Autodesk Inventor part; units mm, degrees
(part 2 of 3)
extrude "Выдавливание11" cut sketch "Эскиз1" against normal blind 6 contours A60 | A65
extrude "Выдавливание12" cut sketch "Эскиз1" against normal blind 4 contours L135 A107 L140 | A107 L135 | L135 A107 L136 L137 L138 L139 L140 | L140 A107 | L135 L136 A107 | A107 L139 L140 | A107 L136 | L139 A107 | L136 L137 A107 | A107 L138 L139 | A107 L137 | L138 A107 | L137 L138 A107 | A45 L144 A42 L143 L215 L141 | L215 A44 L142 A43 | L152 A108 L147 | A108 L152 L151 L150 L149 L148 L147 | L147 A108 | A108 L152 | A108 L148 L147 | L152 L151 A108 | L148 A108 | A108 L151 | A108 L149 L148 | L151 L150 A108 | L149 A108 | A108 L150 | A108 L150 L149 | L153 L219 L155 A46 L156 A49 | A47 L154 A48 L219 | A70 | A71
extrude "Выдавливание16" cut sketch "Эскиз1" against normal blind 2.5 contours L272 A86 L273 L60 L369 L368 L367 | L60 L66 L367 L372 A13 A85 L272 | A133 L72 L74 L73 L62 L280 | L280 A87 L279 A88 L278 A11 L71 L76 L75 L74 A133 | L60 L367 L66 | L62 L73 L78 L77 L278 A90 L277 A89 L280 | A13 L67 L372 L371 L370 A12 L273 A83 L267 L271 A85 | L291 A94 L290 L111 | L111 L290 A92 L289 A93 L292 A91 L291 | L71 L74 L72 | L367 L368 L369 L60 | L60 L369 L68 L370 L67 L372 L66 L367 | L66 L372 L367 | L72 L73 L62 | L66 L372 L67 | L322 A104 L328 A105 L329 A106 L321 L112 | L112 L321 A103 L322 | L74 L75 L76 L71 | L71 L76 L70 L77 L62 L73 L72 L74 | L72 L73 L74 | L60 L68 L369 | L273 A12 L68 L370 L369 L60 | L62 L77 L78 L73 | L67 L370 L371 L372 | L271 L117 L118 L119 L268 A84 L269 A81 L267 | L267 A83 L274 L122 L117 L271 | L71 L70 L76 | L369 L370 L68 | L77 L70 L62 | L370 L68 L67 | L271 L274 L262 L261 L260 L258 L257 L259 L122 L121 L268 L119 L118 L117 | L117 L122 L274 L259 L262 L271 | A11 L278 L62 L70 L77 L76 | L76 L77 L70 | L256 A82 L268 L121 L122 L274 | L274 L259 L257 L258 L260 L261 L262 | L262 L259 L274 | A10 | L116 L98 L115 L97 L251 A80 L252 A77 L250 A79 L239 A78 L95 | L95 L251 L97 L115 L98 L116 | A28 | A29 | A30 | A31 | A32 | A33 | A34 | A35 | L126 L127 L228 A75 L227 A73 L226 A74 L229 A72 L129 L130 L125 | L125 L130 L129 L228 L127 L126 | A38 | A39 | A50 | A51 | L160 L161 L162 L163 L164 L165 | L166 L167 L168 L169 L170 L171 | A52 L175 A53 L174 A54 L173 A55 L172 | A59 L181 A58 L180 A56 L179 A57 L178 | A60 | L187 L188 L189 L190 L191 L192 | A63 L196 A61 L195 A64 L194 A62 L193 | A69 L202 A66 L201 A67 L200 A68 L199 | A65 | L205 L206 L207 L208 L209 L210 | L220 L221 L222 L223 L224 L225 | L232 L234 L236 L235 L233 L231 | L237 L246 L247 L248 L249 L253 | L241 L243 L244 L245 L242 L240 | L254 L263 L264 L265 L266 L270 | L283 L284 L285 L286 L287 L288 | L298 A96 L304 A97 L305 A98 L297 A95 | L295 L299 L301 L306 L300 L296 | L310 A100 L316 A101 L317 A102 L309 A99 | L307 L311 L313 L318 L312 L308 | L319 L323 L325 L330 L324 L320 | A134
sketch "Эскиз3" plane through (0, 0, 4) normal (0, 0, 1) x (1, 0, 0)
  circle A0 centre (0, 55) radius 8 construction
  line L0 (-40.4221, -16.9869) -> (-34.9221, -26.5131)
  line L1 (-47.6314, -27.5) -> (0, 0) construction
  line L2 (-3, 128.25) -> (3, 128.25)
  line L3 (3, 128.25) -> (3, 122.2132)
  line L4 (-3, 122.2132) -> (-3, 128.25)
  line L5 (0, 63) -> (-54.5596, -31.5) construction
  line L6 (14, -6) -> (49, -6) construction
  line L7 (49, 6) -> (14, 6) construction
  line L8 (14, 6) -> (14, -6) construction
  line L9 (48.4771, 7.2527) -> (36.0246, 6.1632) construction
  line L10 (31, 11) -> (37, 11)
  line L11 (49, 1.2755) -> (48.4771, 7.2527) construction
  line L12 (49, 1.2755) -> (36.0246, 6.1632) construction
  line L13 (36.0246, 6.1632) -> (36.5476, 0.186) construction
  line L14 (36.5476, 0.186) -> (48.4771, 7.2527) construction
  line L15 (49, -2.1336) -> (36.5685, -0.827) construction
  line L16 (36.5685, -0.827) -> (35.9413, -6.7941) construction
  line L17 (35.9413, -6.7941) -> (48.3728, -8.1007) construction
  line L18 (49, 11) -> (19, 11)
  line L19 (0, 0) -> (63, 0) construction
  line L20 (14, -6) -> (49, 6) construction
  line L21 (49, -6) -> (14, 6) construction
  line L22 (19, -11) -> (49, -11)
  line L23 (37, -11) -> (31, -11)
  line L24 (48.3728, -8.1007) -> (36.5685, -0.827) construction
  circle A1 centre (0, -34.641) radius 20.7845 construction
  line L25 (31, -18) -> (37, -18)
  line L26 (37, -18) -> (37, -11)
  line L27 (31, -11) -> (31, -18)
  line L28 (54.5596, -31.5) -> (0, 63) construction
  circle A2 centre (0, 0) radius 55.4255 construction
  line L29 (-60.25, 121.25) -> (93.75, 121.25) construction
  line L30 (-60.25, 111.25) -> (93.75, 111.25) construction
  line L31 (-126.25, -126.25) -> (-126.25, 126.25)
  line L32 (-118.25, 74.25) -> (118.75, 74.25) construction
  line L33 (167.75, 130.25) -> (-130.25, 130.25)
  circle A3 centre (0, 0) radius 63
  line L34 (118.75, 59.25) -> (-118.25, 59.25) construction
  circle A4 centre (0, 0) radius 104
  circle A5 centre (0, 0) radius 110.3675
  line L35 (163.75, -126.25) -> (-126.25, -126.25)
  circle A6 centre (0, 0) radius 118.266 construction
  circle A7 centre (0, 0) radius 119.25
  line L36 (-130.25, -130.25) -> (167.75, -130.25)
  line L37 (-130.25, 130.25) -> (-130.25, -130.25)
  circle A8 centre (0, 0) radius 122.25
  line L38 (-126.25, 126.25) -> (163.75, 126.25)
  line L39 (163.75, 126.25) -> (163.75, -126.25)
  line L40 (-3, -128.25) -> (-3, -122.2132)
  line L41 (3, -128.25) -> (-3, -128.25)
  line L42 (3, -122.2132) -> (3, -128.25)
  line L43 (0, -128.25) -> (0, -119.25)
  line L44 (93, -126.25) -> (108, -126.25)
  circle A9 centre (93.75, -116.25) radius 5
  line L45 (-60.25, -111.25) -> (93.75, -111.25) construction
  line L46 (-60.25, -121.25) -> (93.75, -121.25) construction
  line L47 (-128.25, 3) -> (-128.25, -3)
  line L48 (-128.25, -3) -> (-122.2132, -3)
  line L49 (19, 11) -> (19, -11)
  line L50 (0, 0) -> (0, 14.85) construction
  line L51 (-49.5106, -37.2452) -> (-57.0106, -24.2548)
  circle A10 centre (-47.6314, -27.5) radius 2.5
  circle A11 centre (-38.7032, -26.9641) radius 1.5
  line L52 (-33.9221, -28.2452) -> (-57.0106, -24.2548) construction
  line L53 (-35.6542, -29.2452) -> (-49.5106, -37.2452)
  line L54 (167.75, -130.25) -> (167.75, 130.25)
  line L55 (-54.5596, -31.5) -> (54.5596, -31.5) construction
  line L56 (-126.25, -126.25) -> (-126.25, -130.25)
  line L57 (-122.2132, 3) -> (-128.25, 3)
  line L58 (-128.25, 0) -> (-119.25, 0)
  circle A12 centre (-118.25, 66.75) radius 7.5
  circle A13 centre (-42.7032, -20.0359) radius 1.5
  line L59 (-49.5106, -37.2452) -> (-41.4221, -15.2548) construction
  line L60 (-57.0106, -24.2548) -> (-43.1542, -16.2548)
  circle A14 centre (-47.6314, -27.5) radius 8 construction
  line L61 (-116.25, 101.25) -> (-70.25, 101.25) construction
  line L62 (163.75, 116.25) -> (163.75, 100.25)
  line L63 (0, -26.641) -> (0, -25.9661) construction
  circle A15 centre (93.75, 116.25) radius 5
  line L64 (35.6166, 11.7) -> (32.3834, 11.7)
  line L65 (32.3834, 11.7) -> (30.7668, 14.5)
  circle A16 centre (34, 14.5) radius 1.5
  line L66 (37.2332, 14.5) -> (35.6166, 11.7)
  line L67 (37, 11) -> (37, 18)
  arc A17 (37, 18) -> (49, 11) centre (49, 24.7857) ccw
  line L68 (35.9413, -6.7941) -> (49, -2.1336) construction
  line L69 (49, -6) -> (49, 6) construction
  line L70 (48.3728, -8.1007) -> (49, -2.1336) construction
  line L71 (49, -11) -> (49, 11)
  arc A18 (49, -11) -> (37, -18) centre (49, -24.7857) ccw
  circle A19 centre (34, -14.5) radius 1.5
  line L72 (32.3834, -17.3) -> (30.7668, -14.5)
  line L73 (32.3834, -11.7) -> (35.6166, -11.7)
  line L74 (35.6166, -11.7) -> (37.2332, -14.5)
  arc A20 (19, -11) -> (31, -18) centre (31, -4.2143) ccw
  line L75 (37.2332, -14.5) -> (35.6166, -17.3)
  line L76 (35.6166, -17.3) -> (32.3834, -17.3)
  line L77 (30.7668, -14.5) -> (32.3834, -11.7)
  line L78 (31, 18) -> (31, 11)
  arc A21 (31, 18) -> (19, 11) centre (31, 4.2143) ccw
  line L79 (37, 18) -> (31, 18)
  line L80 (32.3834, 17.3) -> (35.6166, 17.3)
  line L81 (35.6166, 17.3) -> (37.2332, 14.5)
  circle A22 centre (118.75, 66.75) radius 7.5
  line L82 (30.7668, 14.5) -> (32.3834, 17.3)
  line L83 (163.75, 126.25) -> (163.75, 130.25)
  line L84 (165.75, 116.25) -> (165.75, 100.25) construction
  line L85 (163.75, 100.25) -> (163.75, 116.25)
  line L86 (36.5476, 0.186) -> (49, 1.2755) construction
  line L87 (0, 0) -> (155.7962, -16.3748) construction
  line L88 (0, 0) -> (156.1718, 0) construction
  line L89 (0, 0) -> (156.3391, 13.6779) construction
  circle A23 centre (130, 40) radius 7.5
  line L90 (130, 47.5) -> (15, 47.5) construction
  line L91 (130, 32.5) -> (15, 32.5) construction
  line L92 (0, 128.25) -> (0, 119.25)
  circle A24 centre (15, 40) radius 7.5
  line L93 (-116.25, -126.25) -> (-70.25, -126.25) construction
  line L94 (-70.25, -106.25) -> (-116.25, -106.25) construction
  line L95 (-116.25, -106.25) -> (-116.25, -126.25) construction
  line L96 (-70.25, -126.25) -> (-70.25, -106.25) construction
  line L97 (-76, -126.25) -> (-61, -126.25)
  circle A25 centre (-60.25, -116.25) radius 5
  line L98 (162.25, -124.75) -> (162.25, -54.75)
  line L99 (112.25, -54.75) -> (112.25, -124.75)
  line L100 (162.25, -54.75) -> (112.25, -54.75)
  line L101 (163.75, -126.25) -> (163.75, -130.25)
  circle A26 centre (159.75, -122.75) radius 1.5
  circle A27 centre (159.75, -56.75) radius 1.5
  circle A28 centre (114.75, -56.75) radius 1.5
  line L102 (112.25, -124.75) -> (162.25, -124.75)
  line L103 (137.25, -89.75) -> (137.25, -86.8436) construction
  line L104 (137.25, -89.75) -> (144.2557, -89.75) construction
  line L105 (144.2557, -89.75) -> (137.25, -89.75) construction
  circle A29 centre (114.75, -122.75) radius 1.5
  line L106 (-126.25, 126.25) -> (-126.25, 130.25)
  line L107 (-70.25, 126.25) -> (-116.25, 126.25) construction
  line L108 (-70.25, 101.25) -> (-70.25, 126.25) construction
  line L109 (-116.25, 126.25) -> (-116.25, 101.25) construction
  circle A30 centre (-60.25, 116.25) radius 5
  circle A31 centre (15.5, -19.141) radius 1.75
  circle A32 centre (-15.5, -19.141) radius 1.75
  line L110 (0, -34.641) -> (5.9719, -34.641)
  line L111 (0, -34.641) -> (0, -30.5774)
  line L112 (21.15, -13.491) -> (-21.15, -13.491)
  circle A33 centre (-15.5, -50.141) radius 1.75
  line L113 (-21.15, -13.491) -> (-21.15, -55.791)
  line L114 (-21.15, -55.791) -> (21.15, -55.791)
  line L115 (21.15, -13.491) -> (-21.15, -55.791) construction
  line L116 (-21.15, -13.491) -> (21.15, -55.791) construction
  line L117 (21.15, -55.791) -> (21.15, -13.491)
  circle A34 centre (15.5, -50.141) radius 1.75
  line L118 (16.5, -13.491) -> (21.15, -18.141)
  line L119 (-16.5, -13.491) -> (-21.15, -18.141)
  line L120 (19, 11) -> (14, 11)
  line L121 (14, 11) -> (14, -11)
  line L122 (14, -11) -> (19, -11)
  line L123 (19, -11) -> (19, 11)
  line L124 (-43.1542, -16.2548) -> (-40.4221, -16.9869)
  line L125 (-35.6542, -29.2452) -> (-34.9221, -26.5131)
  line L126 (34.9221, -26.5131) -> (40.4221, -16.9869)
  line L127 (35.6542, -29.2452) -> (34.9221, -26.5131)
  line L128 (49.5106, -37.2452) -> (35.6542, -29.2452)
  line L129 (57.0106, -24.2548) -> (49.5106, -37.2452)
  line L130 (43.1542, -16.2548) -> (57.0106, -24.2548)
  line L131 (43.1542, -16.2548) -> (40.4221, -16.9869)
  circle A35 centre (42.7032, -20.0359) radius 1.5
  circle A36 centre (38.7032, -26.9641) radius 1.5
  circle A37 centre (47.6314, -27.5) radius 2.5
  circle A38 centre (47.6314, -27.5) radius 8 construction
  line L132 (57.0106, -24.2548) -> (33.9221, -28.2452) construction
  line L133 (41.4221, -15.2548) -> (49.5106, -37.2452) construction
  line L134 (5.5, 43.5) -> (-5.5, 43.5)
  line L135 (7.5, 45.5) -> (5.5, 43.5)
  line L136 (7.5, 61.5) -> (7.5, 45.5)
  line L137 (-7.5, 61.5) -> (7.5, 61.5)
  line L138 (-7.5, 45.5) -> (-7.5, 61.5)
  line L139 (-7.5, 45.5) -> (-5.5, 43.5)
  circle A39 centre (-4, 47) radius 1.5
  circle A40 centre (4, 47) radius 1.5
  circle A41 centre (0, 55) radius 2.5
  circle A42 centre (0, 55) radius 8 construction
  line L140 (-7.5, 61.5) -> (7.5, 43.5) construction
  line L141 (-7.5, 43.5) -> (7.5, 61.5) construction
  line L142 (165.75, 100.25) -> (163.75, 100.25) construction
  line L143 (165.75, 116.25) -> (163.75, 116.25) construction
  line L144 (163.75, -116.25) -> (163.75, -100.25)
  line L145 (165.75, -116.25) -> (163.75, -116.25) construction
  line L146 (165.75, -100.25) -> (163.75, -100.25) construction
  line L147 (165.75, -116.25) -> (165.75, -100.25) construction
  line L148 (163.75, -100.25) -> (163.75, -116.25)
  circle A43 centre (80, 17.5) radius 5.11 projected
  circle A44 centre (80, -17.5) radius 5.11 projected
  circle A45 centre (-80, -17.5) radius 5.11 projected
  circle A46 centre (-80, 17.5) radius 5.11 projected
  line L149 (87.95, 17.5) -> (87.95, -17.5) projected
  arc A47 (72.05, -17.5) -> (87.95, -17.5) centre (80, -17.5) ccw projected
  line L150 (72.05, -17.5) -> (72.05, 17.5) projected
  arc A48 (87.95, 17.5) -> (72.05, 17.5) centre (80, 17.5) ccw projected
  line L151 (-72.05, -17.5) -> (-72.05, 17.5) projected
  line L152 (-87.95, 17.5) -> (-87.95, -17.5) projected
  arc A49 (-72.05, 17.5) -> (-87.95, 17.5) centre (-80, 17.5) ccw projected
  arc A50 (-87.95, -17.5) -> (-72.05, -17.5) centre (-80, -17.5) ccw projected
  line L153 (-102.25, 70.75) -> (-108.25, 70.75) projected
  arc A51 (-102.25, 70.75) -> (-100.25, 72.75) centre (-102.25, 72.75) ccw projected
  line L154 (-100.25, 84.75) -> (-100.25, 72.75) projected
  arc A52 (-100.25, 84.75) -> (-102.25, 86.75) centre (-102.25, 84.75) ccw projected
  line L155 (-108.25, 86.75) -> (-102.25, 86.75) projected
  arc A53 (-102.25, -86.75) -> (-100.25, -84.75) centre (-102.25, -84.75) ccw projected
  line L156 (-108.25, -86.75) -> (-102.25, -86.75) projected
  line L157 (-100.25, -84.75) -> (-100.25, -72.75) projected
  arc A54 (-100.25, -72.75) -> (-102.25, -70.75) centre (-102.25, -72.75) ccw projected
  line L158 (-102.25, -70.75) -> (-108.25, -70.75) projected
  line L159 (-106.25, 84.75) -> (-106.25, 72.75) projected
  arc A55 (-106.25, 84.75) -> (-108.25, 86.75) centre (-108.25, 84.75) ccw projected
  line L160 (-120.25, 86.75) -> (-108.25, 86.75) projected
  arc A56 (-120.25, 86.75) -> (-122.25, 84.75) centre (-120.25, 84.75) ccw projected
  line L161 (-122.25, 72.75) -> (-122.25, 84.75) projected
  arc A57 (-122.25, 72.75) -> (-120.25, 70.75) centre (-120.25, 72.75) ccw projected
  line L162 (-108.25, 70.75) -> (-120.25, 70.75) projected
  arc A58 (-108.25, 70.75) -> (-106.25, 72.75) centre (-108.25, 72.75) ccw projected
  line L163 (-122.25, -84.75) -> (-122.25, -72.75) projected
  arc A59 (-122.25, -84.75) -> (-120.25, -86.75) centre (-120.25, -84.75) ccw projected
  line L164 (-108.25, -86.75) -> (-120.25, -86.75) projected
  arc A60 (-108.25, -86.75) -> (-106.25, -84.75) centre (-108.25, -84.75) ccw projected
  line L165 (-106.25, -72.75) -> (-106.25, -84.75) projected
  arc A61 (-106.25, -72.75) -> (-108.25, -70.75) centre (-108.25, -72.75) ccw projected
  line L166 (-120.25, -70.75) -> (-108.25, -70.75) projected
  arc A62 (-120.25, -70.75) -> (-122.25, -72.75) centre (-120.25, -72.75) ccw projected
  line L167 (-91.95, -17.5) -> (-91.95, 17.5)
  arc A63 (-68.05, 17.5) -> (-91.95, 17.5) centre (-80, 17.5) ccw
  line L168 (-68.05, 17.5) -> (-68.05, -17.5)
  arc A64 (-91.95, -17.5) -> (-68.05, -17.5) centre (-80, -17.5) ccw
  line L169 (68.05, 17.5) -> (68.05, -17.5)
  arc A65 (68.05, -17.5) -> (91.95, -17.5) centre (80, -17.5) ccw
  line L170 (91.95, -17.5) -> (91.95, 17.5)
  arc A66 (91.95, 17.5) -> (68.05, 17.5) centre (80, 17.5) ccw
  line L171 (140.75, -116.25) -> (136.75, -116.25) projected
  arc A67 (134.75, -114.25) -> (136.75, -116.25) centre (136.75, -114.25) ccw projected
  line L172 (134.75, -114.25) -> (134.75, -102.25) projected
  arc A68 (136.75, -100.25) -> (134.75, -102.25) centre (136.75, -102.25) ccw projected
  line L173 (136.75, -100.25) -> (140.75, -100.25) projected
  line L174 (142.75, -100.25) -> (140.75, -100.25) projected
  line L175 (154.75, -100.25) -> (142.75, -100.25) projected
  arc A69 (156.75, -102.25) -> (154.75, -100.25) centre (154.75, -102.25) ccw projected
  line L176 (156.75, -114.25) -> (156.75, -102.25) projected
  arc A70 (154.75, -116.25) -> (156.75, -114.25) centre (154.75, -114.25) ccw projected
  line L177 (142.75, -116.25) -> (154.75, -116.25) projected
  line L178 (142.75, -116.25) -> (140.75, -116.25) projected
  line L179 (154.75, 100.25) -> (142.75, 100.25) projected
  line L180 (142.75, 100.25) -> (140.75, 100.25) projected
  line L181 (136.75, 100.25) -> (140.75, 100.25) projected
  arc A71 (134.75, 102.25) -> (136.75, 100.25) centre (136.75, 102.25) ccw projected
  line L182 (134.75, 114.25) -> (134.75, 102.25) projected
  arc A72 (136.75, 116.25) -> (134.75, 114.25) centre (136.75, 114.25) ccw projected
  line L183 (140.75, 116.25) -> (136.75, 116.25) projected
  line L184 (142.75, 116.25) -> (140.75, 116.25) projected
  line L185 (142.75, 116.25) -> (154.75, 116.25) projected
  arc A73 (156.75, 114.25) -> (154.75, 116.25) centre (154.75, 114.25) ccw projected
  line L186 (156.75, 114.25) -> (156.75, 102.25) projected
  arc A74 (154.75, 100.25) -> (156.75, 102.25) centre (154.75, 102.25) ccw projected
  point P0 (-45.4663, -26.25)
  point P1 (42.5123, 3.7193)
  point P2 (34, 11)
  point P3 (31.5, 0)
  point P4 (34, -11)
  point P5 (31, -14.5)
  point P6 (0, 122.25)
  point P7 (0, -122.25)
  point P8 (-122.25, 0)
  point P9 (-45.4663, -26.25)
  point P10 (42.4707, -4.4638)
  point P11 (31, 14.5)
  point P12 (112.25, -89.75)
  point P13 (137.25, -124.75)
  point P14 (54.5596, -31.5)
  point P15 (45.4663, -26.25)
  point P16 (0, 63)
  point P17 (0, 52.5)
  point P18 (-108.25, -70.75)
  point P19 (-108.25, -86.75)
  point P20 (-108.25, 70.75)
  dimension "d239" = 16
  dimension "d185" = 236.532
  dimension "d186" = 238.5
  dimension "d187" = 290
  dimension "d188" = 3
  dimension "d189" = 6
  dimension "d190" = 4
  dimension "d191" = 208
  dimension "d192" = 220.735
  dimension "d193" = 126
  dimension "d194" = 4
  dimension "d195" = 2
  dimension "d196" = 2
  dimension "d197" = 2
  dimension "d198" = 25
  dimension "d199" = 46
  dimension "d200" = 20
  dimension "d201" = 10
  dimension "d202" = 10
  dimension "d203" = 10
  dimension "d204" = 10
  dimension "d205" = 110.851
  dimension "d206" = 5
  dimension "d207" = 6
  dimension "d211" = 41.569
  dimension "d212" = 12
  dimension "d213" = 35
  dimension "d214" = 6
  dimension "d215" = 12.5
  dimension "d216" = 5
  dimension "d217" = 3
  dimension "d218" = 5.6
  dimension "d219" = 7
  dimension "d220" = 6
  dimension "d222" = 10
  dimension "d223" = 10
  dimension "d224" = 52
  dimension "d225" = 45
  dimension "d226" = 15
  dimension "d227" = 40
  dimension "d228" = 15
  dimension "d229" = 15
  dimension "d230" = 115
  dimension "d231" = 70
  dimension "d232" = 50
  dimension "d233" = 42
  dimension "d234" = 63
  dimension "d235" = 3
  dimension "d236" = 1.5
  dimension "d240" = 4
  dimension "d241" = 18
  dimension "d242" = 15
  dimension "d243" = 3
  dimension "d244" = 2
  dimension "d245" = 2
  dimension "d246" = 5
  dimension "d247" = 237
  dimension "d248" = 42.3
  dimension "d249" = 3.5
  dimension "d250" = 31
  dimension "d251" = 31
  dimension "d252" = 33
  dimension "d253" = 30
  dimension "d254" = 5
  dimension "d255" = 22
  constraints: 308 end point, 42 centre point, 39 point on line, 31 perpendicular, 31 point on circle, 27 parallel, 23 midpoint, 22 vertical alignment, 21 horizontal, 16 tangent, 15 coincident, 13 equal length, 13 symmetric about line, 9 horizontal alignment, 7 vertical, 6 equal radius, 1 collinear, 145 other
  measures "d185" diameter of A6
  measures "d186" diameter of A7
  measures "d187" distance of L31.end L38.end
  measures "d189" distance between parallel lines of L4 L3
  measures "d190" distance between parallel lines of L38 L33
  measures "d191" diameter of A4
  measures "d192" diameter of A5
  measures "d193" diameter of A3
  measures "d194" distance from line of point (-122.25, 0) L31
  measures "d195" distance between parallel lines of L38 L2
  measures "d196" distance between parallel lines of L31 L47
  measures "d197" distance between parallel lines of L35 L41
  measures "d198" distance of L107.end L61.start
  measures "d199" distance of L108.end L107.end
  measures "d200" distance of L94.end L95.end
  measures "d201" distance between parallel lines of L31 L95
  measures "d202" distance between parallel lines of L31 L109
  measures "d203" diameter of A30
  measures "d204" diameter of A15
  measures "d205" diameter of A2
  measures "d206" angle of L88 L89
  measures "d207" angle of L88 L87
  measures "d211" diameter of A1
  measures "d212" distance of L6.end L7.start
  measures "d213" distance of L7.start L8.start
  measures "d214" distance of L11.start L14.end
  measures "d215" distance of L14.end L9.end
  measures "d216" distance between parallel lines of L7 L18
  measures "d217" diameter of A19
  measures "d218" distance between parallel lines of L73 L76
  measures "d219" distance of L23.end L25.start
  measures "d220" distance of L25.start L25.end
  measures "d222" distance from line of L108 A30.centre
  measures "d223" distance from line of L38 A30.centre
  measures "d224" distance between parallel lines of L38 L32
  measures "d225" distance from line of L39 A22.centre
  measures "d226" diameter of A24
  measures "d227" vertical distance of A4.centre A24.centre
  measures "d228" horizontal distance of A4.centre A24.centre
  measures "d229" diameter of A23
  measures "d230" distance of L91.start L91.end
  measures "d231" distance of L98.start L98.end
  measures "d232" distance of L98.end L99.start
  measures "d235" diameter of A29
  measures "d236" distance between parallel lines of L35 L102
  measures "d240" distance edge to line of A10 L51
  measures "d241" distance of L52.end L59.end
  measures "d242" distance of L59.end L52.start
  measures "d243" diameter of A13
  measures "d244" distance edge to line of A13 L0
  measures "d245" distance edge to line of A13 L60
  measures "d246" diameter of A10
  measures "d247" distance of L32.start L32.end
  measures "d248" distance of L114.start L114.end
  measures "d249" diameter of A34
  measures "d250" distance of A31.centre A34.centre
  measures "d251" distance of A32.centre A31.centre
  measures "d252" distance of L119.start L118.start
  measures "d253" distance between parallel lines of L49 L71
  measures "d254" distance between parallel lines of L121 L49
  measures "d255" distance of L22.end L18.start
extrude "Выдавливание17" cut sketch "Эскиз1" against normal through all contours A107 L135 | L135 A107 L136 L137 L138 L139 L140 | L140 A107 | A107 L136 | L139 A107 | A107 L137 | L138 A107 | A108 L152 L151 L150 L149 L148 L147 | L147 A108 | A108 L152 | L148 A108 | A108 L151 | L149 A108 | A108 L150 | A70 | A71
extrude "Выдавливание19" add sketch "Эскиз3" against normal blind 4 separate body contours L0 L125 L53 L51 L60 L124 | L4 L38 L106 L33 L83 L3 L2 | L2 L92 L38 L4 | L2 L3 L38 L92 | L38 L92 A8 L4 | L4 A8 L57 L31 L38 | L38 L3 A8 L92 | A8 L92 A7 L58 | L31 L57 L47 L48 L56 L36 L37 L33 L106 | L38 L39 L35 L42 A8 L3 | A8 L43 A7 L92 | A8 L58 L31 L57 | L31 L58 L47 L57 | L83 L33 L54 L36 L101 L39 | A7 | L58 A7 L43 A8 | A8 L48 L31 L58 | L31 L48 L47 L58 | A8 L40 L35 L31 L48 | L42 L35 L43 A8 | A8 L43 L35 L40 | L35 L40 L41 L42 L101 L36 L56 | L42 L41 L43 L35 | L35 L43 L41 L40 | L78 L65 L64 L66 L67 L10 | L10 L18 L71 L22 L49 | L18 A21 L78 L82 L65 | L67 L66 L81 A17 L18 | L49 L122 L121 L120 | L78 L82 L80 L81 L67 L66 L64 L65 | L65 L82 L78 | L67 L81 L66 | L22 L27 L77 L72 A20 L117 L112 | L79 L67 L81 L80 L82 L78 | A18 L26 L75 L74 L22 | L22 L26 L74 L73 L77 L27 | L112 L117 A20 | A20 L117 L118 L112 | L25 L27 L72 L76 L75 L26 | L77 L73 L74 L26 L75 L76 L72 L27 | L27 L72 L77 | L118 L117 L114 L113 L119 L112 | L74 L75 L26 | L119 L113 L112 | A3 | A4 | A5 | A9 | A10 | A11 | A12 L161 A57 L162 | L162 A57 L161 A12 | A12 L161 A56 L160 A55 L159 A58 L162 | A58 L159 A55 L155 A52 L154 A51 L153 | A13 | A15 | A16 | A19 | A22 | A23 | A24 | A25 | L102 L99 L100 L98 | A26 | A27 | A28 | A29 | A30 | A31 | A32 | A33 | A34 | L126 L131 L130 L129 L128 L127 | A35 | A36 | A37 | L134 L139 L138 L137 L136 L135 | A39 | A40 | A41 | A43 | A44 | A45 | A46 | L149 A47 L150 A48 | A50 L152 A49 L151 | L156 A60 L165 A61 L158 A54 L157 A53 | L164 A59 L163 A62 L166 A61 L165 A60 | L167 A63 L168 A64 | A66 L170 A65 L169 | L171 A67 L172 A68 L173 L174 L175 A69 L176 A70 L177 L178 | L179 L180 L181 A71 L182 A72 L183 L184 L185 A73 L186 A74
extrude "Выдавливание21" cut sketch "Эскиз3" against normal through all contours A43 | A44 | A45 | A46 | L149 A47 L150 A48 | A50 L152 A49 L151 bodies 2
extrude "Выдавливание22" cut sketch "Эскиз1" along normal blind 10 contours A6 | A7 | A10 | A15 | A16 | A17 | A18 | A19 | A20 | A21 | A22 | A23 | A24 | A28 | A29 | A30 | A31 | A32 | A33 | A34 | A35 | A38 | A39 | L135 A107 L140 | A107 L135 | L135 A107 L136 L137 L138 L139 L140 | L140 A107 | L135 L136 A107 | A107 L139 L140 | A107 L136 | L139 A107 | L136 L137 A107 | A107 L138 L139 | A107 L137 | L138 A107 | L137 L138 A107 | A45 L144 A42 L143 L215 L141 | L215 A44 L142 A43 | L152 A108 L147 | A108 L152 L151 L150 L149 L148 L147 | L147 A108 | A108 L152 | A108 L148 L147 | L152 L151 A108 | L148 A108 | A108 L151 | A108 L149 L148 | L151 L150 A108 | L149 A108 | A108 L150 | A108 L150 L149 | L153 L219 L155 A46 L156 A49 | A47 L154 A48 L219 | A50 | A51 | A60 | A65 | A70 | A71 | A134 bodies 2
extrude "Выдавливание23" cut sketch "Эскиз1" against normal blind 6 contours A30 | A31 | A32 | A33 bodies 1
extrude "Выдавливание24" cut sketch "Эскиз1" against normal up to surface (6 mm away) contours A10 | A21 | A22 | A23 | A24 | A28 | A29 | A34 | A35 | A38 | A39 | A50 | A51 | A134 bodies 1
extrude "Выдавливание27" cut sketch "Эскиз3" against normal blind 2 contours L167 A63 L168 A64 | A66 L170 A65 L169 bodies 2
extrude "Выдавливание30" cut sketch "Эскиз1" against normal through all contours A117 | A132 L342 | L342 A132 L343 L344 L345 L346 L347 | L347 A132 | A132 L343 | L346 A132 | A132 L344 | L345 A132 | A124 | A131 L363 L362 L361 L360 L359 L358 | L358 A131 | A131 L363 | L359 A131 | A131 L362 | L360 A131 | A131 L361 bodies 1
extrude "Выдавливание31" cut sketch "Эскиз1" against normal blind 4 contours L334 A121 L335 A120 L336 A123 L337 A122 | A117 | L342 A132 L347 | A132 L342 | L342 A132 L343 L344 L345 L346 L347 | L347 A132 | L342 L343 A132 | A132 L346 L347 | A132 L343 | L346 A132 | L343 L344 A132 | A132 L345 L346 | A132 L344 | L344 L345 A132 | L345 A132 | A129 L353 A130 L352 A127 L351 A128 L350 | A124 | L363 A131 L358 | A131 L363 L362 L361 L360 L359 L358 | L358 A131 | A131 L363 | A131 L359 L358 | L363 L362 A131 | L359 A131 | A131 L362 | A131 L360 L359 | L362 L361 A131 | L360 A131 | A131 L361 L360 | A131 L361 bodies 1
extrude "Выдавливание32" cut sketch "Эскиз1" along normal through all contours L334 A121 L335 A120 L336 A123 L337 A122 | A117 | L342 A132 L347 | A132 L342 | L342 A132 L343 L344 L345 L346 L347 | L347 A132 | L342 L343 A132 | A132 L346 L347 | A132 L343 | L346 A132 | L343 L344 A132 | A132 L345 L346 | A132 L344 | L344 L345 A132 | L345 A132 | A129 L353 A130 L352 A127 L351 A128 L350 | A124 | L363 A131 L358 | A131 L363 L362 L361 L360 L359 L358 | L358 A131 | A131 L363 | A131 L359 L358 | L363 L362 A131 | L359 A131 | A131 L362 | A131 L360 L359 | L362 L361 A131 | L360 A131 | A131 L361 L360 | A131 L361 bodies 2
extrude "Выдавливание33" cut sketch "Эскиз3" against normal blind 2 contours A58 L159 A55 L155 A52 L154 A51 L153 | L156 A60 L165 A61 L158 A54 L157 A53 | L171 A67 L172 A68 L173 L174 L175 A69 L176 A70 L177 L178 | L179 L180 L181 A71 L182 A72 L183 L184 L185 A73 L186 A74 bodies 2
sketch "Эскиз4" plane through (0, 0, 4) normal (0, 0, 1) x (1, 0, 0)
  circle A0 centre (0, 55) radius 8 construction
  line L0 (-40.4221, -16.9869) -> (-34.9221, -26.5131)
  line L1 (-47.6314, -27.5) -> (0, 0) construction
  line L2 (-3, 128.25) -> (3, 128.25)
  line L3 (3, 128.25) -> (3, 122.2132)
  line L4 (-3, 122.2132) -> (-3, 128.25)
  line L5 (0, 63) -> (-54.5596, -31.5) construction
  line L6 (14, -6) -> (49, -6) construction
  line L7 (49, 6) -> (14, 6) construction
  line L8 (14, 6) -> (14, -6) construction
  line L9 (48.4771, 7.2527) -> (36.0246, 6.1632) construction
  line L10 (31, 11) -> (37, 11)
  line L11 (49, 1.2755) -> (48.4771, 7.2527) construction
  line L12 (49, 1.2755) -> (36.0246, 6.1632) construction
  line L13 (36.0246, 6.1632) -> (36.5476, 0.186) construction
  line L14 (36.5476, 0.186) -> (48.4771, 7.2527) construction
  line L15 (49, -2.1336) -> (36.5685, -0.827) construction
  line L16 (36.5685, -0.827) -> (35.9413, -6.7941) construction
  line L17 (35.9413, -6.7941) -> (48.3728, -8.1007) construction
  line L18 (49, 11) -> (19, 11)
  line L19 (0, 0) -> (63, 0) construction
  line L20 (14, -6) -> (49, 6) construction
  line L21 (49, -6) -> (14, 6) construction
  line L22 (19, -11) -> (49, -11)
  line L23 (37, -11) -> (31, -11)
  line L24 (48.3728, -8.1007) -> (36.5685, -0.827) construction
  circle A1 centre (0, -34.641) radius 20.7845 construction
  line L25 (31, -18) -> (37, -18)
  line L26 (37, -18) -> (37, -11)
  line L27 (31, -11) -> (31, -18)
  line L28 (54.5596, -31.5) -> (0, 63) construction
  circle A2 centre (0, 0) radius 55.4255 construction
  line L29 (-70.25, 121.25) -> (93.75, 121.25) construction
  line L30 (-70.25, 111.25) -> (93.75, 111.25) construction
  line L31 (-126.25, -126.25) -> (-126.25, 126.25)
  line L32 (-117.25, 68.25) -> (118.75, 68.25) construction
  line L33 (167.75, 130.25) -> (-130.25, 130.25)
  circle A3 centre (0, 0) radius 63
  line L34 (118.75, 53.25) -> (-117.25, 53.25) construction
  circle A4 centre (0, 0) radius 104
  circle A5 centre (0, 0) radius 110.3675
  line L35 (163.75, -126.25) -> (-126.25, -126.25)
  circle A6 centre (0, 0) radius 118.266 construction
  circle A7 centre (0, 0) radius 119.25
  line L36 (-130.25, -130.25) -> (167.75, -130.25)
  line L37 (-130.25, 130.25) -> (-130.25, -130.25)
  circle A8 centre (0, 0) radius 122.25
  line L38 (-126.25, 126.25) -> (163.75, 126.25)
  line L39 (163.75, 126.25) -> (163.75, -126.25)
  line L40 (-3, -128.25) -> (-3, -122.2132)
  line L41 (3, -128.25) -> (-3, -128.25)
  line L42 (3, -122.2132) -> (3, -128.25)
  line L43 (0, -128.25) -> (0, -119.25)
  line L44 (93, -126.25) -> (108, -126.25)
  circle A9 centre (93.75, -116.25) radius 5
  line L45 (-70.25, -111.25) -> (93.75, -111.25) construction
  line L46 (-70.25, -121.25) -> (93.75, -121.25) construction
  line L47 (-128.25, 3) -> (-128.25, -3)
  line L48 (-128.25, -3) -> (-122.2132, -3)
  line L49 (19, 11) -> (19, -11)
  line L50 (0, 0) -> (0, 14.3794) construction
  line L51 (-49.5106, -37.2452) -> (-57.0106, -24.2548)
  circle A10 centre (-47.6314, -27.5) radius 2.5
  circle A11 centre (-38.7032, -26.9641) radius 1.5
  line L52 (-33.9221, -28.2452) -> (-57.0106, -24.2548) construction
  line L53 (-35.6542, -29.2452) -> (-49.5106, -37.2452)
  line L54 (167.75, -130.25) -> (167.75, 130.25)
  line L55 (-54.5596, -31.5) -> (54.5596, -31.5) construction
  line L56 (-126.25, -126.25) -> (-126.25, -130.25)
  line L57 (-122.2132, 3) -> (-128.25, 3)
  line L58 (-128.25, 0) -> (-119.25, 0)
  circle A12 centre (-117.25, 60.75) radius 7.5
  circle A13 centre (-42.7032, -20.0359) radius 1.5
  line L59 (-49.5106, -37.2452) -> (-41.4221, -15.2548) construction
  line L60 (-57.0106, -24.2548) -> (-43.1542, -16.2548)
  circle A14 centre (-47.6314, -27.5) radius 8 construction
  line L61 (-126.25, 101.25) -> (-80.25, 101.25)
  line L62 (163.75, 116.25) -> (163.75, 100.25)
  line L63 (0, -27.1116) -> (0, -26.4367) construction
  circle A15 centre (93.75, 116.25) radius 5
  line L64 (35.5588, 11.8) -> (32.4412, 11.8)
  line L65 (32.4412, 11.8) -> (30.8823, 14.5)
  circle A16 centre (34, 14.5) radius 1.5
  line L66 (37.1177, 14.5) -> (35.5588, 11.8)
  line L67 (37, 11) -> (37, 18)
  arc A17 (37, 18) -> (49, 11) centre (49, 24.7857) ccw
  line L68 (35.9413, -6.7941) -> (49, -2.1336) construction
  line L69 (49, -6) -> (49, 6) construction
  line L70 (48.3728, -8.1007) -> (49, -2.1336) construction
  line L71 (49, -11) -> (49, 11)
  arc A18 (49, -11) -> (37, -18) centre (49, -24.7857) ccw
  arc A19 (19, -11) -> (31, -18) centre (31, -4.2143) ccw
  line L72 (31, 18) -> (31, 11)
  arc A20 (31, 18) -> (19, 11) centre (31, 4.2143) ccw
  line L73 (37, 18) -> (31, 18)
  line L74 (32.4412, 17.2) -> (35.5588, 17.2)
  line L75 (35.5588, 17.2) -> (37.1177, 14.5)
  circle A21 centre (118.75, 60.75) radius 7.5
  line L76 (30.8823, 14.5) -> (32.4412, 17.2)
  line L77 (163.75, 126.25) -> (163.75, 130.25)
  line L78 (163.75, 100.25) -> (163.75, 116.25)
  line L79 (36.5476, 0.186) -> (49, 1.2755) construction
  line L80 (0, 0) -> (155.7962, -16.3748) construction
  line L81 (0, 0) -> (156.4435, 0) construction
  line L82 (0, 0) -> (156.3391, 13.6779) construction
  circle A22 centre (135, 40) radius 7.5
  line L83 (135, 47.5) -> (25, 47.5) construction
  line L84 (135, 32.5) -> (25, 32.5) construction
  line L85 (0, 128.25) -> (0, 119.25)
  circle A23 centre (25, 40) radius 7.5
  line L86 (-126.25, -126.25) -> (-80.25, -126.25)
  line L87 (-80.25, -101.25) -> (-126.25, -101.25)
  line L88 (-126.25, -101.25) -> (-126.25, -126.25)
  line L89 (-80.25, -126.25) -> (-80.25, -101.25)
  line L90 (-76, -126.25) -> (-61, -126.25)
  circle A24 centre (-70.25, -116.25) radius 5
  line L91 (162.25, -124.75) -> (162.25, -54.75)
  line L92 (112.25, -54.75) -> (112.25, -124.75)
  line L93 (162.25, -54.75) -> (112.25, -54.75)
  line L94 (163.75, -126.25) -> (163.75, -130.25)
  circle A25 centre (159.75, -122.75) radius 1.5
  circle A26 centre (159.75, -56.75) radius 1.5
  circle A27 centre (114.75, -56.75) radius 1.5
  line L95 (112.25, -124.75) -> (162.25, -124.75)
  line L96 (137.25, -89.75) -> (137.25, -87.3142) construction
  line L97 (137.25, -89.75) -> (144.5274, -89.75) construction
  line L98 (144.5274, -89.75) -> (137.25, -89.75) construction
  circle A28 centre (114.75, -122.75) radius 1.5
  line L99 (-126.25, 126.25) -> (-126.25, 130.25)
  line L100 (-80.25, 126.25) -> (-126.25, 126.25)
  line L101 (-80.25, 101.25) -> (-80.25, 126.25)
  line L102 (-126.25, 126.25) -> (-126.25, 101.25)
  circle A29 centre (-70.25, 116.25) radius 5
  circle A30 centre (15.5, -19.141) radius 1.5
  circle A31 centre (-15.5, -19.141) radius 1.5
  line L103 (0, -34.641) -> (5.9719, -34.641)
  line L104 (0, -34.641) -> (0, -31.0481)
  line L105 (21.15, -13.491) -> (-21.15, -13.491)
  circle A32 centre (-15.5, -50.141) radius 1.5
  line L106 (-21.15, -13.491) -> (-21.15, -55.791)
  line L107 (-21.15, -55.791) -> (21.15, -55.791)
  line L108 (21.15, -13.491) -> (-21.15, -55.791) construction
  line L109 (-21.15, -13.491) -> (21.15, -55.791) construction
  line L110 (21.15, -55.791) -> (21.15, -13.491)
  circle A33 centre (15.5, -50.141) radius 1.5
  line L111 (16.5, -13.491) -> (21.15, -18.141)
  line L112 (-16.5, -13.491) -> (-21.15, -18.141)
  line L113 (19, 11) -> (14, 11)
  line L114 (14, 11) -> (14, -11)
  line L115 (14, -11) -> (19, -11)
  line L116 (19, -11) -> (19, 11)
  line L117 (-43.1542, -16.2548) -> (-40.4221, -16.9869)
  line L118 (-35.6542, -29.2452) -> (-34.9221, -26.5131)
  line L119 (34.9221, -26.5131) -> (40.4221, -16.9869)
  line L120 (35.6542, -29.2452) -> (34.9221, -26.5131)
  line L121 (49.5106, -37.2452) -> (35.6542, -29.2452)
  line L122 (57.0106, -24.2548) -> (49.5106, -37.2452)
  line L123 (43.1542, -16.2548) -> (57.0106, -24.2548)
  line L124 (43.1542, -16.2548) -> (40.4221, -16.9869)
  circle A34 centre (42.7032, -20.0359) radius 1.5
  circle A35 centre (38.7032, -26.9641) radius 1.5
  circle A36 centre (47.6314, -27.5) radius 2.5
  circle A37 centre (47.6314, -27.5) radius 8 construction
  line L125 (57.0106, -24.2548) -> (33.9221, -28.2452) construction
  line L126 (41.4221, -15.2548) -> (49.5106, -37.2452) construction
  line L127 (5.5, 43.5) -> (-5.5, 43.5)
  line L128 (7.5, 45.5) -> (5.5, 43.5)
  line L129 (7.5, 61.5) -> (7.5, 45.5)
  line L130 (-7.5, 61.5) -> (7.5, 61.5)
  line L131 (-7.5, 45.5) -> (-7.5, 61.5)
  line L132 (-7.5, 45.5) -> (-5.5, 43.5)
  circle A38 centre (-4, 47) radius 1.5
  circle A39 centre (4, 47) radius 1.5
  circle A40 centre (0, 55) radius 2.5
  circle A41 centre (0, 55) radius 8 construction
  line L133 (-7.5, 61.5) -> (7.5, 43.5) construction
  line L134 (-7.5, 43.5) -> (7.5, 61.5) construction
  line L135 (163.75, -116.25) -> (163.75, -100.25)
  line L136 (163.75, -100.25) -> (163.75, -116.25)
  line L137 (-109.3, 75.8921) -> (-114.25, 73.0342)
  line L138 (-114.25, 73.0342) -> (-119.2, 75.8921)
  line L139 (-119.2, 75.8921) -> (-119.2, 81.6079)
  line L140 (-119.2, 81.6079) -> (-114.25, 84.4658)
  line L141 (-114.25, 84.4658) -> (-109.3, 81.6079)
  line L142 (-109.3, 81.6079) -> (-109.3, 75.8921)
  line L143 (-120.25, 70.75) -> (-108.25, 70.75)
  line L144 (-106.25, 72.75) -> (-106.25, 84.75)
  line L145 (-108.25, 86.75) -> (-120.25, 86.75)
  line L146 (-122.25, 84.75) -> (-122.25, 72.75)
  line L147 (-122.25, 70.75) -> (-106.25, 86.75) construction
  line L148 (-106.25, 70.75) -> (-122.25, 86.75) construction
  arc A42 (-120.25, 86.75) -> (-122.25, 84.75) centre (-120.25, 84.75) ccw
  arc A43 (-108.25, 70.75) -> (-106.25, 72.75) centre (-108.25, 72.75) ccw
  arc A44 (-106.25, 84.75) -> (-108.25, 86.75) centre (-108.25, 84.75) ccw
  arc A45 (-122.25, 72.75) -> (-120.25, 70.75) centre (-120.25, 72.75) ccw
  arc A46 (-122.25, -84.75) -> (-120.25, -86.75) centre (-120.25, -84.75) ccw
  line L149 (-119.2, -75.8921) -> (-119.2, -81.6079)
  line L150 (-109.3, -81.6079) -> (-109.3, -75.8921)
  line L151 (-119.2, -81.6079) -> (-114.25, -84.4658)
  line L152 (-114.25, -84.4658) -> (-109.3, -81.6079)
  line L153 (-108.25, -86.75) -> (-120.25, -86.75)
  line L154 (-114.25, -73.0342) -> (-119.2, -75.8921)
  line L155 (-109.3, -75.8921) -> (-114.25, -73.0342)
  line L156 (-122.25, -84.75) -> (-122.25, -72.75)
  arc A47 (-120.25, -70.75) -> (-122.25, -72.75) centre (-120.25, -72.75) ccw
  line L157 (-120.25, -70.75) -> (-108.25, -70.75)
  line L158 (-106.25, -70.75) -> (-122.25, -86.75) construction
  line L159 (-122.25, -70.75) -> (-106.25, -86.75) construction
  arc A48 (-106.25, -72.75) -> (-108.25, -70.75) centre (-108.25, -72.75) ccw
  line L160 (-106.25, -72.75) -> (-106.25, -84.75)
  arc A49 (-108.25, -86.75) -> (-106.25, -84.75) centre (-108.25, -84.75) ccw
  line L161 (-126.25, 101.25) -> (-80.25, 101.25)
  circle A50 centre (-114.75, 95.75) radius 1.5
  circle A51 centre (-91.75, 95.75) radius 1.5
  line L162 (-112.05, 97.3088) -> (-112.05, 94.1912)
  line L163 (-112.05, 94.1912) -> (-114.75, 92.6323)
  line L164 (-114.75, 92.6323) -> (-117.45, 94.1912)
  line L165 (-117.45, 94.1912) -> (-117.45, 97.3088)
  line L166 (-117.45, 97.3088) -> (-114.75, 98.8677)
  line L167 (-114.75, 98.8677) -> (-112.05, 97.3088)
  line L168 (-91.75, 98.8677) -> (-89.05, 97.3088)
  line L169 (-89.05, 97.3088) -> (-89.05, 94.1912)
  line L170 (-89.05, 94.1912) -> (-91.75, 92.6323)
  line L171 (-91.75, 92.6323) -> (-94.45, 94.1912)
  line L172 (-94.45, 94.1912) -> (-94.45, 97.3088)
  line L173 (-94.45, 97.3088) -> (-91.75, 98.8677)
  line L174 (-117.5, 91) -> (-112, 91)
  line L175 (-110, 93) -> (-110, 98.5)
  line L176 (-112, 100.5) -> (-117.5, 100.5)
  line L177 (-119.5, 98.5) -> (-119.5, 93)
  line L178 (-119.5, 91) -> (-110, 100.5) construction
  line L179 (-110, 91) -> (-119.5, 100.5) construction
  line L180 (-89, 100.5) -> (-94.5, 100.5)
  line L181 (-96.5, 98.5) -> (-96.5, 93)
  line L182 (-94.5, 91) -> (-89, 91)
  line L183 (-87, 93) -> (-87, 98.5)
  line L184 (-87, 100.5) -> (-96.5, 91) construction
  line L185 (-96.5, 100.5) -> (-87, 91) construction
  arc A52 (-119.5, 93) -> (-117.5, 91) centre (-117.5, 93) ccw
  arc A53 (-117.5, 100.5) -> (-119.5, 98.5) centre (-117.5, 98.5) ccw
  arc A54 (-110, 98.5) -> (-112, 100.5) centre (-112, 98.5) ccw
  arc A55 (-112, 91) -> (-110, 93) centre (-112, 93) ccw
  arc A56 (-96.5, 93) -> (-94.5, 91) centre (-94.5, 93) ccw
  arc A57 (-94.5, 100.5) -> (-96.5, 98.5) centre (-94.5, 98.5) ccw
  arc A58 (-89, 91) -> (-87, 93) centre (-89, 93) ccw
  arc A59 (-87, 98.5) -> (-89, 100.5) centre (-89, 98.5) ccw
  line L186 (-126.25, -101.25) -> (-80.25, -101.25)
  line L187 (-80.25, -101.25) -> (-80.25, -100.25)
  line L188 (-90.25, -90.25) -> (-116.25, -90.25)
  circle A60 centre (-91.75, -95.75) radius 1.5
  line L189 (-91.75, -92.6323) -> (-89.05, -94.1912)
  line L190 (-89.05, -94.1912) -> (-89.05, -97.3088)
  line L191 (-89.05, -97.3088) -> (-91.75, -98.8677)
  line L192 (-91.75, -98.8677) -> (-94.45, -97.3088)
  line L193 (-94.45, -97.3088) -> (-94.45, -94.1912)
  line L194 (-94.45, -94.1912) -> (-91.75, -92.6323)
  line L195 (-94.5, -100.5) -> (-89, -100.5)
  line L196 (-87, -98.5) -> (-87, -93)
  line L197 (-89, -91) -> (-94.5, -91)
  line L198 (-96.5, -93) -> (-96.5, -98.5)
  line L199 (-96.5, -100.5) -> (-87, -91) construction
  line L200 (-87, -100.5) -> (-96.5, -91) construction
  arc A61 (-94.5, -91) -> (-96.5, -93) centre (-94.5, -93) ccw
  arc A62 (-89, -100.5) -> (-87, -98.5) centre (-89, -98.5) ccw
  arc A63 (-96.5, -98.5) -> (-94.5, -100.5) centre (-94.5, -98.5) ccw
  arc A64 (-87, -93) -> (-89, -91) centre (-89, -93) ccw
  line L201 (-117.5, -100.5) -> (-112, -100.5)
  line L202 (-110, -98.5) -> (-110, -93)
  line L203 (-112, -91) -> (-117.5, -91)
  line L204 (-119.5, -93) -> (-119.5, -98.5)
  line L205 (-119.5, -100.5) -> (-110, -91) construction
  line L206 (-110, -100.5) -> (-119.5, -91) construction
  circle A65 centre (-114.75, -95.75) radius 1.5
  line L207 (-112.05, -94.1912) -> (-112.05, -97.3088)
  line L208 (-112.05, -97.3088) -> (-114.75, -98.8677)
  line L209 (-114.75, -98.8677) -> (-117.45, -97.3088)
  line L210 (-117.45, -97.3088) -> (-117.45, -94.1912)
  line L211 (-117.45, -94.1912) -> (-114.75, -92.6323)
  line L212 (-114.75, -92.6323) -> (-112.05, -94.1912)
  line L213 (-126.25, -100.25) -> (-126.25, -101.25)
  arc A66 (-117.5, -91) -> (-119.5, -93) centre (-117.5, -93) ccw
  arc A67 (-110, -93) -> (-112, -91) centre (-112, -93) ccw
  arc A68 (-112, -100.5) -> (-110, -98.5) centre (-112, -98.5) ccw
  arc A69 (-119.5, -98.5) -> (-117.5, -100.5) centre (-117.5, -98.5) ccw
  line L214 (-108.25, 86.75) -> (-102.25, 86.75)
  line L215 (-100.25, 84.75) -> (-100.25, 72.75)
  line L216 (-102.25, 70.75) -> (-108.25, 70.75)
  line L217 (-108.25, 70.75) -> (-108.25, 86.75)
  line L218 (-108.25, -86.75) -> (-102.25, -86.75)
  line L219 (-100.25, -84.75) -> (-100.25, -72.75)
  line L220 (-102.25, -70.75) -> (-108.25, -70.75)
  line L221 (-108.25, -70.75) -> (-108.25, -86.75)
  circle A70 centre (-114.25, 78.75) radius 3
  circle A71 centre (-114.25, -78.75) radius 3
  arc A72 (-9.7, 44.25) -> (-7.7, 42.25) centre (-7.7, 44.25) ccw
  line L222 (6.7, 45.4412) -> (4, 43.8823)
  line L223 (6.7, 48.5588) -> (6.7, 45.4412)
  line L224 (-7.7, 42.25) -> (7.7, 42.25)
  line L225 (9.7, 44.25) -> (9.7, 49.75)
  line L226 (4, 43.8823) -> (1.3, 45.4412)
  line L227 (4, 50.1177) -> (6.7, 48.5588)
  arc A73 (9.7, 49.75) -> (7.7, 51.75) centre (7.7, 49.75) ccw
  line L228 (1.3, 45.4412) -> (1.3, 48.5588)
  line L229 (-9.7, 49.75) -> (-9.7, 44.25)
  line L230 (1.3, 48.5588) -> (4, 50.1177)
  arc A74 (-7.7, 51.75) -> (-9.7, 49.75) centre (-7.7, 49.75) ccw
  line L231 (7.7, 51.75) -> (-7.7, 51.75)
  arc A75 (7.7, 42.25) -> (9.7, 44.25) centre (7.7, 44.25) ccw
  line L232 (0, 42.25) -> (0, 44.9705) construction
  line L233 (-4, 50.1177) -> (-6.7, 48.5588)
  line L234 (-6.7, 45.4412) -> (-4, 43.8823)
  line L235 (-6.7, 48.5588) -> (-6.7, 45.4412)
  line L236 (-1.3, 45.4412) -> (-1.3, 48.5588)
  line L237 (-4, 43.8823) -> (-1.3, 45.4412)
  line L238 (-1.3, 48.5588) -> (-4, 50.1177)
  circle A76 centre (-4, 47) radius 1.5
  line L239 (-42.7032, -16.9182) -> (-40.0032, -18.4771)
  arc A77 (-40.4396, -14.4566) -> (-43.1716, -13.7246) centre (-42.1716, -15.4566) ccw
  line L240 (-36.5896, -21.125) -> (-38.9456, -22.4853) construction
  arc A78 (-40.9668, -32.5434) -> (-38.2348, -33.2754) centre (-39.2348, -31.5434) ccw
  line L241 (-38.2348, -33.2754) -> (-33.4716, -30.5254)
  line L242 (-38.7032, -30.0818) -> (-36.0032, -28.5229)
  arc A79 (-33.4716, -30.5254) -> (-32.7396, -27.7934) centre (-34.4716, -28.7934) ccw
  line L243 (-41.4032, -28.5229) -> (-38.7032, -30.0818)
  line L244 (-36.0032, -28.5229) -> (-36.0032, -25.4053)
  line L245 (-41.4032, -25.4053) -> (-41.4032, -28.5229)
  line L246 (-38.7032, -23.8464) -> (-41.4032, -25.4053)
  line L247 (-36.0032, -25.4053) -> (-38.7032, -23.8464)
  line L248 (-40.0032, -18.4771) -> (-40.0032, -21.5947)
  line L249 (-40.0032, -21.5947) -> (-42.7032, -23.1536)
  line L250 (-42.7032, -23.1536) -> (-45.4032, -21.5947)
  line L251 (-45.4032, -21.5947) -> (-45.4032, -18.4771)
  line L252 (-32.7396, -27.7934) -> (-40.4396, -14.4566)
  line L253 (-48.6668, -19.2066) -> (-40.9668, -32.5434)
  arc A80 (-47.9348, -16.4746) -> (-48.6668, -19.2066) centre (-46.9348, -18.2066) ccw
  line L254 (-43.1716, -13.7246) -> (-47.9348, -16.4746)
  line L255 (-45.4032, -18.4771) -> (-42.7032, -16.9182)
  line L256 (36.0032, -28.5229) -> (36.0032, -25.4053)
  arc A81 (32.7396, -27.7934) -> (33.4716, -30.5254) centre (34.4716, -28.7934) ccw
  line L257 (36.5896, -21.125) -> (38.9456, -22.4853) construction
  arc A82 (48.6668, -19.2066) -> (47.9348, -16.4746) centre (46.9348, -18.2066) ccw
  line L258 (47.9348, -16.4746) -> (43.1716, -13.7246)
  line L259 (45.4032, -18.4771) -> (42.7032, -16.9182)
  arc A83 (43.1716, -13.7246) -> (40.4396, -14.4566) centre (42.1716, -15.4566) ccw
  line L260 (45.4032, -21.5947) -> (45.4032, -18.4771)
  line L261 (42.7032, -16.9182) -> (40.0032, -18.4771)
  line L262 (42.7032, -23.1536) -> (45.4032, -21.5947)
  line L263 (40.0032, -21.5947) -> (42.7032, -23.1536)
  line L264 (40.0032, -18.4771) -> (40.0032, -21.5947)
  line L265 (36.0032, -25.4053) -> (38.7032, -23.8464)
  line L266 (38.7032, -23.8464) -> (41.4032, -25.4053)
  line L267 (41.4032, -25.4053) -> (41.4032, -28.5229)
  line L268 (41.4032, -28.5229) -> (38.7032, -30.0818)
  line L269 (40.4396, -14.4566) -> (32.7396, -27.7934)
  line L270 (40.9668, -32.5434) -> (48.6668, -19.2066)
  arc A84 (38.2348, -33.2754) -> (40.9668, -32.5434) centre (39.2348, -31.5434) ccw
  line L271 (33.4716, -30.5254) -> (38.2348, -33.2754)
  line L272 (38.7032, -30.0818) -> (36.0032, -28.5229)
  line L273 (37.9143, -22.8306) -> (26.5604, -16.2754)
  line L274 (25.8284, -13.5434) -> (29.0857, -7.9015)
  line L275 (31.8178, -7.1694) -> (43.1716, -13.7246)
  line L276 (43.1716, -13.7246) -> (37.9143, -22.8306)
  line L277 (37.9143, -22.8306) -> (30.0857, -6.1694) construction
  line L278 (24.8284, -15.2754) -> (43.1716, -13.7246) construction
  line L279 (34, -14.5) -> (37.8782, -16.7391) construction
  line L280 (34, -14.5) -> (34.9387, -12.8741) construction
  line L281 (30.8823, -14.5) -> (32.4412, -11.8)
  line L282 (32.4412, -11.8) -> (35.5588, -11.8)
  line L283 (35.5588, -11.8) -> (37.1177, -14.5)
  line L284 (37.1177, -14.5) -> (35.5588, -17.2)
  line L285 (35.5588, -17.2) -> (32.4412, -17.2)
  line L286 (32.4412, -17.2) -> (30.8823, -14.5)
  circle A85 centre (34, -14.5) radius 1.5
  arc A86 (25.8284, -13.5434) -> (26.5604, -16.2754) centre (27.5604, -14.5434) ccw
  arc A87 (31.8178, -7.1694) -> (29.0857, -7.9015) centre (30.8178, -8.9015) ccw
  line L287 (31.25, 9.75) -> (36.75, 9.75)
  line L288 (38.75, 11.75) -> (38.75, 17.25)
  line L289 (36.75, 19.25) -> (31.25, 19.25)
  line L290 (29.25, 17.25) -> (29.25, 11.75)
  line L291 (29.25, 9.75) -> (38.75, 19.25) construction
  line L292 (38.75, 9.75) -> (29.25, 19.25) construction
  arc A88 (31.25, 19.25) -> (29.25, 17.25) centre (31.25, 17.25) ccw
  arc A89 (38.75, 17.25) -> (36.75, 19.25) centre (36.75, 17.25) ccw
  arc A90 (29.25, 11.75) -> (31.25, 9.75) centre (31.25, 11.75) ccw
  arc A91 (36.75, 9.75) -> (38.75, 11.75) centre (36.75, 11.75) ccw
  arc A92 (12.75, -14.391) -> (10.75, -16.391) centre (12.75, -16.391) ccw
  line L293 (12.8, -17.5822) -> (15.5, -16.0233)
  line L294 (12.8, -20.6998) -> (12.8, -17.5822)
  line L295 (10.75, -16.391) -> (10.75, -21.891)
  line L296 (18.25, -14.391) -> (12.75, -14.391)
  line L297 (15.5, -16.0233) -> (18.2, -17.5822)
  line L298 (15.5, -22.2587) -> (12.8, -20.6998)
  arc A93 (20.25, -16.391) -> (18.25, -14.391) centre (18.25, -16.391) ccw
  line L299 (18.2, -17.5822) -> (18.2, -20.6998)
  line L300 (10.75, -23.891) -> (20.25, -14.391) construction
  line L301 (20.25, -23.891) -> (10.75, -14.391) construction
  line L302 (20.25, -21.891) -> (20.25, -16.391)
  line L303 (12.75, -23.891) -> (18.25, -23.891)
  line L304 (18.2, -20.6998) -> (15.5, -22.2587)
  arc A94 (18.25, -23.891) -> (20.25, -21.891) centre (18.25, -21.891) ccw
  arc A95 (10.75, -21.891) -> (12.75, -23.891) centre (12.75, -21.891) ccw
  line L305 (-20.25, -47.391) -> (-20.25, -52.891)
  line L306 (-18.2, -51.6998) -> (-18.2, -48.5822)
  arc A96 (-18.25, -45.391) -> (-20.25, -47.391) centre (-18.25, -47.391) ccw
  line L307 (-15.5, -53.2587) -> (-18.2, -51.6998)
  line L308 (-18.2, -48.5822) -> (-15.5, -47.0233)
  line L309 (-12.8, -48.5822) -> (-12.8, -51.6998)
  line L310 (-12.8, -51.6998) -> (-15.5, -53.2587)
  line L311 (-18.25, -54.891) -> (-12.75, -54.891)
  line L312 (-15.5, -47.0233) -> (-12.8, -48.5822)
  line L313 (-12.75, -45.391) -> (-18.25, -45.391)
  line L314 (-10.75, -52.891) -> (-10.75, -47.391)
  arc A97 (-12.75, -54.891) -> (-10.75, -52.891) centre (-12.75, -52.891) ccw
  line L315 (-20.25, -54.891) -> (-10.75, -45.391) construction
  line L316 (-10.75, -54.891) -> (-20.25, -45.391) construction
  arc A98 (-10.75, -47.391) -> (-12.75, -45.391) centre (-12.75, -47.391) ccw
  arc A99 (-20.25, -52.891) -> (-18.25, -54.891) centre (-18.25, -52.891) ccw
  line L317 (10.75, -47.391) -> (10.75, -52.891)
  line L318 (12.8, -51.6998) -> (12.8, -48.5822)
  arc A100 (12.75, -45.391) -> (10.75, -47.391) centre (12.75, -47.391) ccw
  line L319 (15.5, -53.2587) -> (12.8, -51.6998)
  line L320 (12.8, -48.5822) -> (15.5, -47.0233)
  line L321 (18.2, -48.5822) -> (18.2, -51.6998)
  line L322 (18.2, -51.6998) -> (15.5, -53.2587)
  line L323 (12.75, -54.891) -> (18.25, -54.891)
  line L324 (15.5, -47.0233) -> (18.2, -48.5822)
  line L325 (18.25, -45.391) -> (12.75, -45.391)
  line L326 (20.25, -52.891) -> (20.25, -47.391)
  arc A101 (18.25, -54.891) -> (20.25, -52.891) centre (18.25, -52.891) ccw
  line L327 (10.75, -54.891) -> (20.25, -45.391) construction
  line L328 (20.25, -54.891) -> (10.75, -45.391) construction